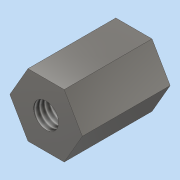
# Autodesk Inventor part: CouplingNutThread_5_40
Saved by Autodesk Inventor 2017 (Build 210142000, 142)
## iProperties
Created: 2016-11-13
Part Number: CouplingNutThread_5_40
Material: Stainless Steel
Document SubType Name: Modeling
Designer: techn
Density: 8 g/cm^3
Appearance: Semi-Polished
Author: techn
Autodesk Inventor part; units mm, degrees
ref_plane "YZ Plane" through (0, 0, 0) normal (1, 0, 0) x (0, 1, 0)
ref_plane "XZ Plane" through (0, 0, 0) normal (0, 1, 0) x (-1, 0, 0)
ref_plane "XY Plane" through (0, 0, 0) normal (0, 0, 1) x (1, 0, 0)
sketch "Sketch1" plane through (0, 0, 0) normal (0, 0, 1) x (1, 0, 0)
  line L0 (-4.5827, 0) -> (-2.2914, 3.9687)
  line L1 (-2.2914, 3.9687) -> (2.2914, 3.9687)
  line L2 (2.2914, 3.9687) -> (4.5827, 0)
  line L3 (4.5827, 0) -> (2.2914, -3.9688)
  line L4 (2.2914, -3.9688) -> (-2.2914, -3.9688)
  line L5 (-2.2914, -3.9688) -> (-4.5827, 0)
  circle A0 centre (0, 0) radius 1.5875
  dimension "d0" = 7.9375
  dimension "d1" = 3.175
  constraints: 12 end point, 2 coincident, 1 centre point, 13 other
  measures "d0" distance between parallel lines of L4 L1
  measures "d1" diameter of A0
extrude "Extrusion1" add sketch "Sketch1" against normal blind 11.1125
thread "Thread1" size "5-40 UNC" class "2B" standard "ANSI Unified Screw Threads" full length
body "Solid1"
